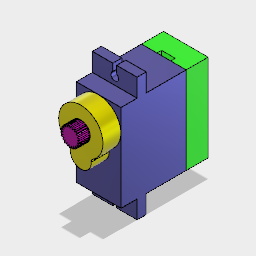
FS90R (Autodesk Fusion 360 design; units mm, degrees)
Autodesk Fusion 360 part; units mm, degrees
sketch "Sketch1" plane through (0, 0, 0) normal (0, 0, 1) x (1, 0, 0)
  line L0 (5.9, 10.7) -> (5.9, -21.9)
  line L1 (-5.9, -21.9) -> (-5.9, 10.7)
  line L2 (0, 18.2992) -> (0, 8.3637)
  line L3 (-0.4974, 10.7) -> (-0.4974, 8.7675)
  line L4 (0.4974, 10.7) -> (0.4974, 8.7675)
  arc A0 (-0.4974, 8.7675) -> (0.4974, 8.7675) centre (0, 7.9) ccw
  line L5 (-5.9, 10.7) -> (-0.4974, 10.7)
  line L6 (0.4974, 10.7) -> (5.9, 10.7)
  line L7 (-8.8231, -5.6) -> (-15.4878, -5.6)
  line L8 (0, -29.4992) -> (0, -19.5637)
  line L9 (-5.9, -21.9) -> (-0.4974, -21.9)
  arc A1 (0.4974, -19.9675) -> (-0.4974, -19.9675) centre (0, -19.1) ccw
  line L10 (0.4974, -21.9) -> (5.9, -21.9)
  line L11 (0.4974, -21.9) -> (0.4974, -19.9675)
  line L12 (-0.4974, -21.9) -> (-0.4974, -19.9675)
  line L13 (5.9, -21.9) -> (0.4974, -21.9)
  line L14 (-0.4974, -21.9) -> (-5.9, -21.9)
  line L15 (-5.9, 5.9) -> (5.9, 5.9)
  line L16 (-5.9, -17.1) -> (5.9, -17.1)
  circle A2 centre (0, 0) radius 5.9
  dimension "d3" = 5.9
  dimension "d4" = 5.9
  dimension "d7" = 32.6
  dimension "d8" = 2
  dimension "d9" = 2.8
  dimension "d12" = 16.3
  dimension "d13" = 4.8
  measures "d3" distance of A2.centre L1
  measures "d4" distance of A2.centre L0
  measures "d7" distance of L0.start L0.end
  measures "d8" diameter of A0
  measures "d9" distance of A0.centre L5
  measures "d12" distance of L5 L7
  measures "d13" distance of L6 L15
extrude "Extrude1" add sketch "Sketch1" along normal blind 4.25 contours L0 L15 A2 | A2 | L0 L1 L16 A2 | L1 L15 A2 makes body 1
extrude "Extrude2" add sketch "Sketch1" against normal blind 2.4 contours L0 L1 L3 L4 A0 L5 L6 L15 | L0 L1 L9 A1 L10 L11 L12 L13 L14 L16 bodies 1
sketch "Sketch2" plane through (0, 0, 4.25) normal (0, 0, 1) x (1, 0, 0)
  line L0 (-5.9, 5.9) -> (-5.9, -17.1)
  line L1 (-5.9, -17.1) -> (5.9, -17.1)
  line L2 (5.9, -17.1) -> (5.9, 5.9)
  line L3 (5.9, 5.9) -> (-5.9, 5.9)
extrude "Extrude3" add sketch "Sketch2" 1 faces at (-1.9667, -9.4333, 4.25) against normal blind 17.2 on bodies 1 bodies 1
sketch "Sketch4" plane through (0, 0, 4.25) normal (0, 0, 1) x (1, 0, 0)
  line L0 (-5.9, 5.9) -> (-5.9, -17.1)
  line L1 (-5.9, -17.1) -> (5.9, -17.1)
  line L2 (5.9, -17.1) -> (5.9, 5.9)
  line L3 (5.9, 5.9) -> (-5.9, 5.9)
  circle A0 centre (0, 0) radius 2.5
  arc A1 (-2.7433, -5.8081) -> (2.7433, -5.8081) centre (0, -6) ccw
  arc A2 (3.1947, -4.9006) -> (-3.1947, -4.9006) centre (0, 0) ccw
  arc A3 (3.1947, -4.9006) -> (2.7433, -5.8081) centre (3.7409, -5.7383) ccw
  arc A4 (-2.7433, -5.8081) -> (-3.1947, -4.9006) centre (-3.7409, -5.7383) ccw
  dimension "d21" = 5
  dimension "d22" = 5.5
  dimension "d23" = 11.7
  dimension "d24" = 6
  dimension "d25" = 1
  dimension "d26" = 1
  measures "d21" diameter of A0
  measures "d22" diameter of A1
  measures "d23" diameter of A2
  measures "d24" distance of A1.centre A0.centre
  measures "d25" radius of A3
  measures "d26" radius of A4
extrude "Extrude4" add sketch "Sketch4" along normal blind 7.5 separate body contours A0 makes body 2
extrude "Extrude5" add sketch "Sketch4" along normal blind 4.7 separate body contours A1 A2 A3 A4 makes body 3
sketch "Sketch5" plane through (0, 0, 11.75) normal (0, 0, 1) x (1, 0, 0)
  circle A0 centre (0, 0) radius 2.5
  line L0 (-0.0048, 1.9281) -> (0.2004, 2.492)
  line L1 (0, 0) -> (0, 0.9431)
  line L2 (0.0048, 1.9281) -> (-0.2004, 2.492)
  arc A1 (0.2004, 2.492) -> (-0.2004, 2.492) centre (0, 0) ccw
  line L3 (-0.5729, 1.8411) -> (-0.543, 2.4403)
  arc A2 (-0.543, 2.4403) -> (-0.926, 2.3222) centre (0, 0) ccw
  line L4 (-0.5638, 1.8439) -> (-0.926, 2.3222)
  line L5 (-1.0901, 1.5904) -> (-1.2382, 2.1719)
  arc A3 (-1.2382, 2.1719) -> (-1.5694, 1.946) centre (0, 0) ccw
  line L6 (-1.0822, 1.5958) -> (-1.5694, 1.946)
  line L7 (-1.5105, 1.1984) -> (-1.8233, 1.7104)
  arc A4 (-1.8233, 1.7104) -> (-2.0733, 1.397) centre (0, 0) ccw
  line L8 (-1.5045, 1.2059) -> (-2.0733, 1.397)
  line L9 (-1.7966, 0.7) -> (-2.2465, 1.097)
  arc A5 (-2.2465, 1.097) -> (-2.3929, 0.7238) centre (0, 0) ccw
  line L10 (-1.7931, 0.7089) -> (-2.3929, 0.7238)
  line L11 (-1.9231, 0.1393) -> (-2.47, 0.3861)
  arc A6 (-2.47, 0.3861) -> (-2.5, -0.0136) centre (0, 0) ccw
  line L12 (-1.9224, 0.1489) -> (-2.5, -0.0136)
  line L13 (-1.8787, -0.4337) -> (-2.4741, -0.3591)
  arc A7 (-2.4741, -0.3591) -> (-2.3849, -0.7499) centre (0, 0) ccw
  line L14 (-1.8809, -0.4244) -> (-2.3849, -0.7499)
  line L15 (-1.6674, -0.9682) -> (-2.2583, -1.0724)
  arc A8 (-2.2583, -1.0724) -> (-2.0579, -1.4196) centre (0, 0) ccw
  line L16 (-1.6722, -0.9599) -> (-2.0579, -1.4196)
  line L17 (-1.308, -1.4167) -> (-1.8419, -1.6904)
  arc A9 (-1.8419, -1.6904) -> (-1.548, -1.9631) centre (0, 0) ccw
  line L18 (-1.315, -1.4102) -> (-1.548, -1.9631)
  line L19 (-0.8323, -1.7393) -> (-1.2618, -2.1582)
  arc A10 (-1.2618, -2.1582) -> (-0.9006, -2.3321) centre (0, 0) ccw
  line L20 (-0.8409, -1.7351) -> (-0.9006, -2.3321)
  line L21 (-0.2826, -1.9073) -> (-0.5696, -2.4342)
  arc A11 (-0.5696, -2.4342) -> (-0.1732, -2.494) centre (0, 0) ccw
  line L22 (-0.2921, -1.9059) -> (-0.1732, -2.494)
  line L23 (0.2921, -1.9059) -> (0.1732, -2.494)
  arc A12 (0.1732, -2.494) -> (0.5696, -2.4342) centre (0, 0) ccw
  line L24 (0.2826, -1.9073) -> (0.5696, -2.4342)
  line L25 (0.8409, -1.7351) -> (0.9006, -2.3321)
  arc A13 (0.9006, -2.3321) -> (1.2618, -2.1582) centre (0, 0) ccw
  line L26 (0.8323, -1.7393) -> (1.2618, -2.1582)
  line L27 (1.315, -1.4102) -> (1.548, -1.9631)
  arc A14 (1.548, -1.9631) -> (1.8419, -1.6904) centre (0, 0) ccw
  line L28 (1.308, -1.4167) -> (1.8419, -1.6904)
  line L29 (1.6722, -0.9599) -> (2.0579, -1.4196)
  arc A15 (2.0579, -1.4196) -> (2.2583, -1.0724) centre (0, 0) ccw
  line L30 (1.6674, -0.9682) -> (2.2583, -1.0724)
  line L31 (1.8809, -0.4244) -> (2.3849, -0.7499)
  arc A16 (2.3849, -0.7499) -> (2.4741, -0.3591) centre (0, 0) ccw
  line L32 (1.8787, -0.4337) -> (2.4741, -0.3591)
  line L33 (1.9224, 0.1489) -> (2.5, -0.0136)
  arc A17 (2.5, -0.0136) -> (2.47, 0.3861) centre (0, 0) ccw
  line L34 (1.9231, 0.1393) -> (2.47, 0.3861)
  line L35 (1.7931, 0.7089) -> (2.3929, 0.7238)
  arc A18 (2.3929, 0.7238) -> (2.2465, 1.097) centre (0, 0) ccw
  line L36 (1.7966, 0.7) -> (2.2465, 1.097)
  line L37 (1.5045, 1.2059) -> (2.0733, 1.397)
  arc A19 (2.0733, 1.397) -> (1.8233, 1.7104) centre (0, 0) ccw
  line L38 (1.5105, 1.1984) -> (1.8233, 1.7104)
  line L39 (1.0822, 1.5958) -> (1.5694, 1.946)
  arc A20 (1.5694, 1.946) -> (1.2382, 2.1719) centre (0, 0) ccw
  line L40 (1.0901, 1.5904) -> (1.2382, 2.1719)
  line L41 (0.5638, 1.8439) -> (0.926, 2.3222)
  arc A21 (0.926, 2.3222) -> (0.543, 2.4403) centre (0, 0) ccw
  line L42 (0.5729, 1.8411) -> (0.543, 2.4403)
  dimension "d31" = 20
  dimension "d33" = 360
  dimension "d36" = 0.6
  measures "d31" angle of L0 L1
  measures "d36" distance of L0.start L0.end
extrude "Extrude7" cut sketch "Sketch5" against normal blind 2.8 contours A0 L33 A17 L34 | A0 L35 A18 L36 | A0 L31 A16 L32 | A0 L37 A19 L38 | A0 L29 A15 L30 | A0 L39 A20 L40 | A0 L27 A14 L28 | A0 L41 A21 L42 | A0 L25 A13 L26 | A0 L0 L2 A1 | A0 L23 A12 L24 | A0 L3 A2 L4 | A0 L21 A11 L22 | A0 L5 A3 L6 | A0 L19 A10 L20 | A0 L7 A4 L8 | A0 L17 A9 L18 | A0 L9 A5 L10 | A0 L15 A8 L16 | A0 L11 A6 L12 | A0 L13 A7 L14 bodies 2
sketch "Sketch6" plane through (0, 0, -12.95) normal (0, 0, -1) x (-1, 0, 0)
  line L0 (5.9, 5.9) -> (-5.9, 5.9)
  line L1 (-5.9, 5.9) -> (-5.9, -17.1)
  line L2 (-5.9, -17.1) -> (5.9, -17.1)
  line L3 (5.9, -17.1) -> (5.9, 5.9)
extrude "Extrude8" add sketch "Sketch6" along normal blind 5.8 separate body makes body 4
extrude "Extrude6" cut sketch "Sketch5" against normal blind 2.8 contours A0 L33 A17 L34 | A0 L35 A18 L36 | A0 L31 A16 L32 | A0 L37 A19 L38 | A0 L29 A15 L30 | A0 L39 A20 L40 | A0 L27 A14 L28 | A0 L41 A21 L42 | A0 L25 A13 L26 | A0 L0 L2 A1 | A0 L23 A12 L24 | A0 L3 A2 L4 | A0 L21 A11 L22 | A0 L5 A3 L6 | A0 L19 A10 L20 | A0 L7 A4 L8 | A0 L17 A9 L18 | A0 L9 A5 L10 | A0 L15 A8 L16 | A0 L11 A6 L12 | A0 L13 A7 L14 bodies 2
ref_plane "WorkPlane1" through (0, -5.6, -4.35) normal (-1, 0, 0) x (0, 1, 0)
sketch "Sketch7" plane through (0, 5.9, 0) normal (0, 1, 0) x (-1, 0, 0)
  line L0 (5.9, -12.95) -> (-5.9, -12.95)
  line L1 (-5.9, -12.95) -> (-5.9, -18.75)
  line L2 (-5.9, -18.75) -> (5.9, -18.75)
  line L3 (5.9, -18.75) -> (5.9, -12.95)
  line L4 (1.8, -14.15) -> (-1.8, -14.15)
  line L5 (-1.8, -14.15) -> (-1.8, -12.95)
  line L6 (-1.8, -12.95) -> (1.8, -12.95)
  line L7 (1.8, -12.95) -> (1.8, -14.15)
  line L8 (0, -14.67) -> (0, 5.97)
  dimension "d41" = 1.2
  dimension "d42" = 3.6
  dimension "d43" = 1.8
  measures "d41" distance of L4.end L5.end
  measures "d42" distance of L4.start L4.end
  measures "d43" distance of L7 L8
extrude "Extrude9" cut sketch "Sketch7" against normal blind 10 contours L0 L4 L6 L7 L8 | L0 L4 L5 L6 L8 bodies 4
equation "d3 = ( 11.8 / 2 ) * 1 mm"
equation "d4 = d3"
equation "d9 = ( ( 32.6 - 27 ) / 2 ) * 1 mm"
equation "d12 = d7 / 2"
equation "d13 = ( ( 32.6 - 23 ) / 2 ) * 1 mm"
equation "d43 = d42 / 2"
